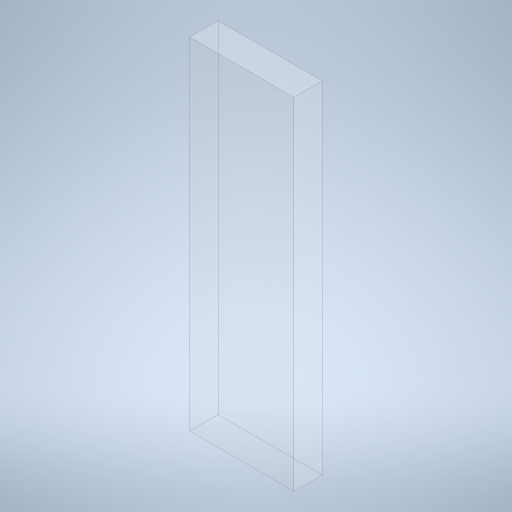
# Autodesk Inventor part: base_bateria2
Saved by Autodesk Inventor 2023 (Build 270158000, 158)
## iProperties
Created: 2023-06-07
Part Number: base_bateria2
Material: Cristal
Document SubType Name: Modeling
Designer: sergi
Density: 2.18 g/cm^3
Appearance: Claro - Ligero
Author: sergi
Autodesk Inventor part; units mm, degrees
ref_plane "YZ Plane" through (0, 0, 0) normal (1, 0, 0) x (0, 1, 0)
ref_plane "XZ Plane" through (0, 0, 0) normal (0, 1, 0) x (-1, 0, 0)
ref_plane "XY Plane" through (0, 0, 0) normal (0, 0, 1) x (1, 0, 0)
sketch "Boceto1" plane through (0, 0, 0) normal (0, 1, 0) x (-1, 0, 0)
  line L0 (-5.5, -1.5) -> (5.5, -1.5)
  line L1 (5.5, -1.5) -> (5.5, 1.5)
  line L2 (5.5, 1.5) -> (-5.5, 1.5)
  line L3 (-5.5, 1.5) -> (-5.5, -1.5)
  line L4 (-5.5, -1.5) -> (5.5, 1.5) construction
  line L5 (5.5, -1.5) -> (-5.5, 1.5) construction
  point P0 (0, 0)
  dimension "d0" = 11
  dimension "d1" = 3
  constraints: 12 end point, 2 midpoint, 2 parallel, 1 horizontal, 1 perpendicular
  measures "d0" distance of L2.end L1.end
  measures "d1" distance of L0.end L1.end
extrude "Extrusión1" add sketch "Boceto1" along normal blind 36
